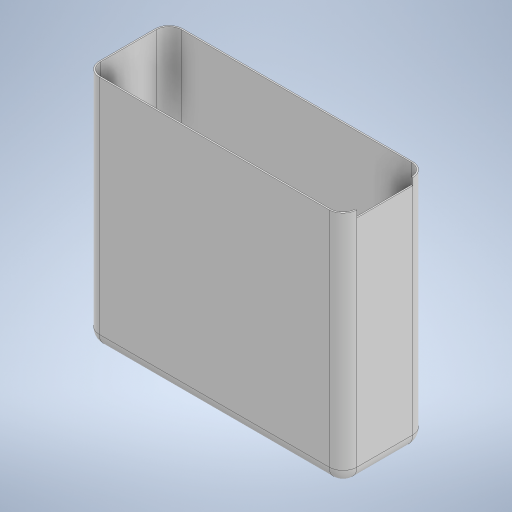
# Autodesk Inventor part: Down_Case
Saved by Autodesk Inventor 2024 (Build 280153000, 153)
## iProperties
Created: 2023-11-21
Part Number: Down_Case
Material: Generic
Document SubType Name: Modeling
Designer: renan
Density: 1 g/cm^3
Appearance: Default
Author: renan
Autodesk Inventor part; units mm, degrees
ref_plane "YZ Plane" through (0, 0, 0) normal (1, 0, 0) x (0, 1, 0)
ref_plane "XZ Plane" through (0, 0, 0) normal (0, 1, 0) x (-1, 0, 0)
ref_plane "XY Plane" through (0, 0, 0) normal (0, 0, 1) x (1, 0, 0)
sketch "Sketch1" plane through (0, 0, 0) normal (0, 1, 0) x (-1, 0, 0)
  line L0 (0, 0) -> (37, 0)
  line L1 (37, 0) -> (37, -12)
  line L2 (37, -12) -> (0, -12)
  line L3 (0, -12) -> (0, 0)
  dimension "d0" = 12
  dimension "d1" = 37
  constraints: 8 end point, 2 parallel, 1 horizontal, 1 perpendicular
  measures "d0" distance of L0.end L1.end
  measures "d1" distance of L1.end L2.end
extrude "Extrusion1" add sketch "Sketch1" along normal blind 34
fillet "Fillet1" radius 2 8 edges at (0, 17, 0) (0, 17, -12) (-37, 17, 0) (-37, 17, -12) (-18.5, 0, 0) (-18.5, 0, -12) (0, 0, -6) (-37, 0, -6)
shell "Shell1" thickness 0.2 removed faces 1 at (-24, 34, -4)
sketch "Sketch2" plane through (0, 2, -10) normal (1, 0, 0) x (0, 0, -1)
  line L0 (0, 32) -> (-8, 32) projected
  line L1 (0, 32) -> (0, 0) projected
  line L2 (-8, 32) -> (0, 32)
  line L3 (0, 32) -> (0, 31)
  line L4 (0, 31) -> (-8, 31)
  line L5 (-8, 31) -> (-8, 32)
  point P0 (-10, -2)
  dimension "d6" = 1
  constraints: 8 end point, 2 parallel, 1 horizontal, 1 perpendicular, 1 point on line
  measures "d6" distance of L4.end L0.end
extrude "Extrusion2" cut sketch "Sketch2" against normal blind 10
body "Solid1"
